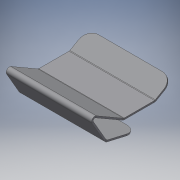
# Autodesk Inventor part: Lamiera pinza
Saved by Autodesk Inventor 2018 (Build 220112000, 112)
## iProperties
Created: 2020-05-30
Part Number: Lamiera pinza
Material: Generico
Document SubType Name: Lamiera
Designer: Francesco
Density: 1 g/cm^3
Sheet Metal Rule: Default_mm
Appearance: Default
Author: Francesco
Autodesk Inventor part; units mm, degrees
ref_plane "YZ Plane" through (0, 0, 0) normal (1, 0, 0) x (0, 1, 0)
ref_plane "XZ Plane" through (0, 0, 0) normal (0, 1, 0) x (-1, 0, 0)
ref_plane "XY Plane" through (0, 0, 0) normal (0, 0, 1) x (1, 0, 0)
sketch "Schizzo1" plane through (0, 0, 0) normal (0, 0, 1) x (1, 0, 0)
  line L0 (-40, 15) -> (40, 15)
  line L1 (40, 15) -> (40, -15)
  line L2 (40, -15) -> (-40, -15)
  line L3 (-40, -15) -> (-40, 15)
  line L4 (-40, 15) -> (40, -15) construction
  line L5 (40, 15) -> (-40, -15) construction
  point P0 (0, 0)
  dimension "d0" = 80
  dimension "d1" = 30
  measures "d0" distance of L1.end L2.end
  measures "d1" distance of L0.end L1.end
extrude "Piano1" add sketch "Schizzo1" along normal blind 1.5
sketch "Schizzo2" plane through (40, -14.25, 1.299) normal (0, -0.5, -0.8660254) x (1, 0, 0)
  line L0 (-80, 0) -> (0, 0)
  line L1 (0, 0) -> (0, 30)
  line L2 (0, 30) -> (-80, 30)
  line L3 (-80, 30) -> (-80, 0)
  constraints: 6 end point, 1 horizontal, 1 perpendicular, 1 vertical
edge flange "Flangia1" height 30 angle 30 thickness 1.5 bend radius 1.5 thickness toward (0, -0.5, -0.8660254) relief straight relief width 1.5 relief depth 0.75 edges at (0, -15, 1.5) wall of the first edge with corners at (-40, -14.25, 1.299) (40, -14.25, 1.299) (40, -40.2308, 16.299) (-40, -40.2308, 16.299)
bend "Piega (Bend)1"
corner "Angolo1"
sketch "Schizzo3" plane through (-40, 14.25, 1.299) normal (0, 0.5, -0.8660254) x (-1, 0, 0)
  line L0 (-80, 0) -> (0, 0)
  line L1 (0, 0) -> (0, 20)
  line L2 (0, 20) -> (-80, 20)
  line L3 (-80, 20) -> (-80, 0)
  constraints: 6 end point, 1 horizontal, 1 perpendicular, 1 vertical
edge flange "Flangia2" height 20 angle 30 thickness 1.5 bend radius 1.5 thickness toward (0, 0.5, -0.8660254) relief straight relief width 1.5 relief depth 0.75 edges at (0, 15, 1.5) wall of the first edge with corners at (40, 14.25, 1.299) (-40, 14.25, 1.299) (-40, 31.5705, 11.299) (40, 31.5705, 11.299)
bend "Piega (Bend)2"
corner "Angolo2"
sketch "Schizzo4" plane through (-40, -43.0298, 12.951) normal (0, -0.8660254, -0.5) x (1, 0, 0)
  line L0 (80, 0) -> (0, 0)
  line L1 (0, 0) -> (0, -23.8038)
  line L2 (0, -23.8038) -> (80, -23.8038)
  line L3 (80, -23.8038) -> (80, 0)
  constraints: 6 end point, 1 horizontal, 1 perpendicular, 1 vertical
edge flange "Flangia3" height 35 angle 150 thickness 1.5 bend radius 1.5 thickness toward (0, -0.8660254, -0.5) relief straight relief width 1.5 relief depth 0.75 edges at (0, -40.9808, 15) wall of the first edge with corners at (40, -43.0298, 12.951) (-40, -43.0298, 12.951) (-40, -31.1279, -7.6638) (40, -31.1279, -7.6638)
bend "Piega (Bend)3"
corner "Angolo3"
sketch "Schizzo6" plane through (-40, -30.1663, -8.3753) normal (0, -0.2249511, -0.9743701) x (1, 0, 0)
  line L0 (80, 0) -> (0, 0)
  line L1 (0, 0) -> (0, -28.6956)
  line L2 (0, -28.6956) -> (80, -28.6956)
  line L3 (80, -28.6956) -> (80, 0)
  constraints: 6 end point, 1 horizontal, 1 perpendicular, 1 vertical
edge flange "Flangia5" height 30 angle 47 thickness 1.5 bend radius 1.5 thickness toward (0, -0.2249511, -0.9743701) relief straight relief width 1.5 relief depth 0.75 edges at (0, -31.1279, -7.6638) wall of the first edge with corners at (40, -30.1663, -8.3753) (-40, -30.1663, -8.3753) (-40, -2.2062, -14.8304) (40, -2.2062, -14.8304)
bend "Piega (Bend)5"
corner "Angolo5"
sketch "Schizzo7" plane through (40, -2.5436, -16.292) normal (0, -0.2249511, -0.9743701) x (-1, 0, 0)
  line L0 (80, 0) -> (80, -28.6956) projected
  line L1 (0, 0) -> (80, 0) projected
  point P0 (40, -1.1865)
  point P1 (40, -14.3478)
  point P2 (80, -14.3478)
  point P3 (40, 0)
  constraints: 2 midpoint, 1 horizontal alignment, 1 vertical alignment
hole "Foro1" at (0, -16.5236, -13.0644) direction (0, 0.2249511, 0.9743701) diameter 10 depth 1.5 tip angle 118
fillet "Arrotondamento angolo1" radius 10 4 edges at (40, 31.9455, 10.6495) (-40, 31.9455, 10.6495) (40, -2.3749, -15.5612) (-40, -2.3749, -15.5612)
equation "\"d58\" = Spessore"
equation "\"d2\" = Spessore"
equation "\"d3\" = LarghezzaScaricoPiega"
equation "\"d4\" = ProfonditàScaricoPiega"
equation "\"d5\" = ResiduoMinimo"
equation "\"d6\" = RaggioTransizione"
equation "\"d9\" = RaggioPiega"
equation "\"d10\" = DimensioniScaricoAngolo"
equation "\"d11\" = DimensioneGioco"
equation "\"d12\" = Dimensione_raggio_Jacobi"
equation "\"d13\" = LarghezzaScaricoPiega"
equation "\"d14\" = ProfonditàScaricoPiega"
equation "\"d15\" = ResiduoMinimo"
equation "\"d16\" = RaggioTransizione"
equation "\"d19\" = RaggioPiega"
equation "\"d20\" = DimensioniScaricoAngolo"
equation "\"d21\" = DimensioneGioco"
equation "\"d22\" = Dimensione_raggio_Jacobi"
equation "\"d23\" = LarghezzaScaricoPiega"
equation "\"d24\" = ProfonditàScaricoPiega"
equation "\"d25\" = ResiduoMinimo"
equation "\"d26\" = RaggioTransizione"
equation "\"d29\" = RaggioPiega"
equation "\"d30\" = DimensioniScaricoAngolo"
equation "\"d31\" = DimensioneGioco"
equation "\"d32\" = Dimensione_raggio_Jacobi"
equation "\"d43\" = LarghezzaScaricoPiega"
equation "\"d44\" = ProfonditàScaricoPiega"
equation "\"d45\" = ResiduoMinimo"
equation "\"d46\" = RaggioTransizione"
equation "\"d49\" = RaggioPiega"
equation "\"d50\" = DimensioniScaricoAngolo"
equation "\"d51\" = DimensioneGioco"
equation "\"d52\" = Dimensione_raggio_Jacobi"
equation "\"RaggioPiega\" = Spessore"
equation "\"LarghezzaScaricoPiega\" = Spessore"
equation "\"ProfonditàScaricoPiega\" = 0.5 * Spessore"
equation "\"DimensioniScaricoAngolo\" = 4 * Spessore"
equation "\"ResiduoMinimo\" = 2 * Spessore"
equation "\"RaggioTransizione\" = RaggioPiega"
equation "\"Dimensione_raggio_Jacobi\" = RaggioPiega"
equation "\"DimensioneGioco\" = Spessore"
equation "\"Spessore\" = 1.5"
